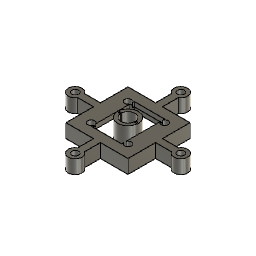
AS5600_MountingFrame v2 (Autodesk Fusion 360 design; units mm, degrees)
Autodesk Fusion 360 part; units mm, degrees
sketch "AS5600" plane through (0, 0, 0) normal (0, 0, 1) x (1, 0, 0)
  line L0 (-8.6, 11.35) -> (8.6, 11.35)
  line L1 (11.6, 8.35) -> (11.6, -8.35)
  line L2 (8.6, -11.35) -> (-8.6, -11.35)
  line L3 (-11.6, -8.35) -> (-11.6, 8.35)
  line L4 (-8, 8) -> (8, 8) construction
  line L5 (8, 8) -> (8, -8) construction
  line L6 (8, -8) -> (-8, -8) construction
  line L7 (-8, -8) -> (-8, 8) construction
  circle A0 centre (-8, 8) radius 1.5
  circle A1 centre (8, 8) radius 1.5
  circle A2 centre (-8, -8) radius 1.5
  circle A3 centre (8, -8) radius 1.5
  arc A4 (-8.6, 11.35) -> (-11.6, 8.35) centre (-8.6, 8.35) ccw
  arc A5 (11.6, 8.35) -> (8.6, 11.35) centre (8.6, 8.35) ccw
  arc A6 (-11.6, -8.35) -> (-8.6, -11.35) centre (-8.6, -8.35) ccw
  arc A7 (8.6, -11.35) -> (11.6, -8.35) centre (8.6, -8.35) ccw
  point P0 (11.6, 11.35)
  point P1 (11.6, -11.35)
  dimension "d6" = 23.2
  dimension "d7" = 22.7
  dimension "d8" = 11.35
  dimension "d10" = 8
  dimension "d11" = 8
  dimension "d12" = 8
  dimension "d13" = 8
  dimension "d14" = 3
  dimension "d15" = 3
  dimension "d16" = 3
  dimension "d17" = 3
  dimension "d18" = 3
  dimension "d19" = 3
  dimension "d20" = 3
  dimension "d21" = 3
  dimension "d22" = 11.6
  constraint horizontal L0
  constraint vertical L1
  constraint horizontal L2
  constraint vertical L3
  constraint horizontal L4
  constraint vertical L5
  constraint horizontal L6
  constraint vertical L7
  constraint coincident L4.start L7.end
  constraint coincident L4.end L5.start
  constraint coincident L6.end L7.start
  constraint coincident L5.end L6.start
  constraint tangent L0 A4
  constraint tangent L3 A4
  constraint coincident P0 L0
  constraint coincident P0 L1
  constraint tangent L0 A5
  constraint tangent L1 A5
  constraint tangent L2 A6
  constraint tangent L3 A6
  constraint coincident P1 L1
  constraint coincident P1 L2
  constraint tangent L1 A7
  constraint tangent L2 A7
  measures "d6" distance of L1 L3
  measures "d7" distance of P0 P1
  measures "d8" distance of L2 origin
  measures "d10" distance of origin L7
  measures "d11" distance of origin L5
  measures "d12" distance of origin L4
  measures "d13" distance of L6 origin
  measures "d14" diameter of A0
  measures "d15" diameter of A1
  measures "d16" diameter of A2
  measures "d17" diameter of A3
  measures "d18" radius of A4
  measures "d19" radius of A5
  measures "d20" radius of A6
  measures "d21" radius of A7
  measures "d22" distance of L1 origin
sketch "Sketch3" plane through (0, 0, 0) normal (0, 0, 1) x (1, 0, 0)
  circle A0 centre (0, 0) radius 23 construction
  circle A1 centre (23, 0) radius 1.5
  line L0 (0, 0) -> (23, 0) construction
  circle A2 centre (23, 0) radius 3
  line L1 (-13.5, 13.5) -> (13.5, 13.5)
  line L2 (13.5, 13.5) -> (13.5, -13.5)
  line L3 (13.5, -13.5) -> (-13.5, -13.5)
  line L4 (-13.5, -13.5) -> (-13.5, 13.5)
  line L5 (-6.6, 9.35) -> (6.6, 9.35)
  line L6 (6.6, 9.35) -> (6.6, -9.35)
  line L7 (6.6, -9.35) -> (-6.6, -9.35)
  line L8 (-6.6, -9.35) -> (-6.6, 9.35)
  line L9 (-11.6, -8.35) -> (-11.6, 8.35)
  line L10 (11.6, 8.35) -> (11.6, -8.35)
  line L11 (8.6, -11.35) -> (-8.6, -11.35)
  line L12 (-8.6, 11.35) -> (8.6, 11.35)
  line L13 (13.5, 1.5) -> (20.4019, 1.5)
  line L14 (13.5, -1.5) -> (20.4019, -1.5)
  circle A3 centre (0, 23) radius 3
  circle A4 centre (0, 23) radius 1.5
  line L15 (1.5, 13.5) -> (1.5, 20.4019)
  line L16 (-1.5, 13.5) -> (-1.5, 20.4019)
  circle A5 centre (-23, 0) radius 3
  circle A6 centre (-23, 0) radius 1.5
  line L17 (-13.5, 1.5) -> (-20.4019, 1.5)
  line L18 (-13.5, -1.5) -> (-20.4019, -1.5)
  circle A7 centre (0, -23) radius 3
  circle A8 centre (0, -23) radius 1.5
  line L19 (-1.5, -13.5) -> (-1.5, -20.4019)
  line L20 (1.5, -13.5) -> (1.5, -20.4019)
  circle A9 centre (8, 8) radius 1.5
  circle A10 centre (-8, 8) radius 1.5
  circle A11 centre (-8, -8) radius 1.5
  circle A12 centre (8, -8) radius 1.5
  dimension "d23" = 46
  dimension "d24" = 3
  dimension "d25" = 6
  dimension "d26" = 13.5
  dimension "d27" = 13.5
  dimension "d28" = 13.5
  dimension "d29" = 13.5
  dimension "d30" = 5
  dimension "d31" = 5
  dimension "d32" = 2
  dimension "d33" = 2
  dimension "d34" = 1.5
  dimension "d35" = 1.5
  dimension "d37" = 360
  constraint coincident A0.centre L0.start
  constraint coincident A0 A1.centre
  constraint coincident A1.centre L0.end
  constraint horizontal L0
  constraint concentric A1 A2
  constraint horizontal L1
  constraint vertical L2
  constraint horizontal L3
  constraint vertical L4
  constraint horizontal L5
  constraint vertical L6
  constraint horizontal L7
  constraint vertical L8
  constraint coincident L2 L13.start
  constraint coincident A2 L13.end
  constraint perpendicular L2 L13
  constraint coincident L2 L14.start
  constraint coincident A2 L14.end
  constraint perpendicular L2 L14
  measures "d23" diameter of A0
  measures "d24" diameter of A1
  measures "d25" diameter of A2
  measures "d26" distance of L2 A0.centre
  measures "d27" distance of L4 A0.centre
  measures "d28" distance of L1 A0.centre
  measures "d29" distance of L3 A0.centre
  measures "d30" distance of L8 L9
  measures "d31" distance of L6 L10
  measures "d32" distance of L7 L11
  measures "d33" distance of L5 L12
  measures "d34" distance of L0 L13
  measures "d35" distance of L0 L14
extrude "Extrude2" add sketch "Sketch3" along normal blind 6 makes body 1
sketch "Sketch4" plane through (0, 0, 0) normal (0, 0, 1) x (1, 0, 0)
  line L0 (-8.6, 11.35) -> (8.6, 11.35)
  line L1 (-11.6, -8.35) -> (-11.6, 8.35)
  arc A0 (-8.6, 11.35) -> (-11.6, 8.35) centre (-8.6, 8.35) ccw
  arc A1 (-11.6, -8.35) -> (-8.6, -11.35) centre (-8.6, -8.35) ccw
  line L2 (8.6, -11.35) -> (-8.6, -11.35)
  arc A2 (8.6, -11.35) -> (11.6, -8.35) centre (8.6, -8.35) ccw
  line L3 (11.6, 8.35) -> (11.6, -8.35)
  arc A3 (11.6, 8.35) -> (8.6, 11.35) centre (8.6, 8.35) ccw
  arc A4 (8.6, -11.55) -> (11.8, -8.35) centre (8.6, -8.35) ccw
  line L4 (11.8, 8.35) -> (11.8, -8.35)
  arc A5 (11.8, 8.35) -> (8.6, 11.55) centre (8.6, 8.35) ccw
  line L5 (-8.6, 11.55) -> (8.6, 11.55)
  arc A6 (-8.6, 11.55) -> (-11.8, 8.35) centre (-8.6, 8.35) ccw
  line L6 (-11.8, -8.35) -> (-11.8, 8.35)
  arc A7 (-11.8, -8.35) -> (-8.6, -11.55) centre (-8.6, -8.35) ccw
  line L7 (8.6, -11.55) -> (-8.6, -11.55)
  dimension "d42" = -0.2
extrude "Extrude3" cut sketch "Sketch4" along normal blind 4 contours L0 L1 A0 A1 L2 A2 L3 A3 | A4 L4 A5 L5 A6 L6 A7 L7 bodies 1
sketch "Sketch1" plane through (0, 0, 0) normal (0, 0, 1) x (1, 0, 0) in component "MagnetHolder1"
  circle A0 centre (0, 0) radius 2.2
  circle A1 centre (0, 0) radius 4.5
  circle A2 centre (0, 0) radius 1.95
  dimension "d45" = 4.4
  dimension "d46" = 9
  dimension "d47" = 3.9
  constraint coincident A0.centre A1.centre
  measures "d45" diameter of A0
  measures "d46" diameter of A1
  measures "d47" diameter of A2
extrude "Extrude1" add sketch "Sketch1" along normal blind 4.5 separate body contours A1 makes body 2 in component "MagnetHolder1"
extrude "Extrude2'" add sketch "Sketch1" along normal blind 2.5 contours A0 bodies 2 in component "MagnetHolder1"
sketch "Sketch2" plane through (0, 0, 0) normal (0, 0, 1) x (1, 0, 0) in component "MagnetHolder1"
  line L0 (-3, 0.5) -> (3, 0.5)
  line L1 (3, 0.5) -> (3, -0.5)
  line L2 (3, -0.5) -> (-3, -0.5)
  line L3 (-3, -0.5) -> (-3, 0.5)
  dimension "d52" = 3
  dimension "d53" = 3
  dimension "d54" = 0.5
  dimension "d55" = 0.5
  constraint horizontal L0
  constraint vertical L1
  constraint horizontal L2
  constraint vertical L3
  measures "d52" distance of L3 origin
  measures "d53" distance of L1 origin
  measures "d54" distance of L0 origin
  measures "d55" distance of L2 origin
extrude "Extrude3'" cut sketch "Sketch2" along normal blind 7.5 bodies 2 in component "MagnetHolder1"
sketch "Sketch1 (2)" plane through (0, 0, 0) normal (0, 0, 1) x (1, 0, 0) in component "MagnetHolder2"
  circle A0 centre (0, 0) radius 3.05
  circle A1 centre (0, 0) radius 2.1
  circle A2 centre (0, 0) radius 4.5
  circle A3 centre (0, 0) radius 1.9
  dimension "d58" = 6.1
  dimension "d59" = 4.2
  dimension "d60" = 9
  dimension "d65" = 3.8
  constraint coincident A0.centre A1.centre
  constraint concentric A0 A1
  measures "d58" diameter of A0
  measures "d59" diameter of A1
  measures "d60" diameter of A2
  measures "d65" diameter of A3
extrude "Extrude1'" add sketch "Sketch1 (2)" along normal blind 8 separate body contours A2 makes body 3 in component "MagnetHolder2"
extrude "Extrude2''" add sketch "Sketch1 (2)" along normal blind 2.5 contours A0 bodies 3 in component "MagnetHolder2"
extrude "Extrude3''" add sketch "Sketch1 (2)" along normal blind 2.5 and the other way blind -2 contours A1 bodies 3 in component "MagnetHolder2"
sketch "Sketch2 (2)" plane through (0, 0, 0) normal (0, 0, 1) x (1, 0, 0) in component "MagnetHolder2"
  line L0 (4, 0.2804) -> (-4, 0.2804)
  line L1 (-4, 0.2804) -> (-4, -0.2948)
  line L2 (-4, -0.2948) -> (4, -0.2948)
  line L3 (4, -0.2948) -> (4, 0.2804)
  dimension "d70" = 4
  dimension "d71" = 4
  constraint horizontal L0
  constraint vertical L1
  constraint horizontal L2
  constraint vertical L3
  measures "d70" distance of L1 origin
  measures "d71" distance of L3 origin
extrude "Extrude4" cut sketch "Sketch2 (2)" along normal blind 9.5 bodies 3 in component "MagnetHolder2"
component "MagnetHolder1" placed x (1, 0, 0) y (0, 1, 0) z (0, 0, 1) at (0, 0, 0)
component "MagnetHolder2" placed x (1, 0, 0) y (0, 1, 0) z (0, 0, 1) at (0, 0, 0)
equation "d8 = ( 22.7 / 2 ) * 1 mm"
named bodies: "AS5600_MountingFrame", "AS5600MagnetHolder1", "AS5600MagentHolder2"
